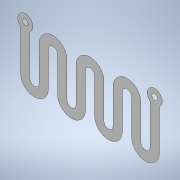
# Autodesk Inventor part: sensor-0002-001
Saved by Autodesk Inventor 2020.1 (Build 241239000, 239)
## iProperties
Created: 2024-03-28
Part Number: sensor-0002-001
Material: Generic
Document SubType Name: Modeling
Designer: MiguelBarbosa
Density: 1 g/cm^3
Appearance: Default
Author: MiguelBarbosa
Autodesk Inventor part; units mm, degrees
ref_plane "YZ Plane" through (0, 0, 0) normal (1, 0, 0) x (0, 1, 0)
ref_plane "XZ Plane" through (0, 0, 0) normal (0, 1, 0) x (-1, 0, 0)
ref_plane "XY Plane" through (0, 0, 0) normal (0, 0, 1) x (1, 0, 0)
sketch "Sketch1" plane through (0, 0, 0) normal (0, 0, 1) x (1, 0, 0)
  circle A0 centre (-2800, 1250) radius 325 construction
  line L0 (-2800, 1250) -> (-2800, -750) construction
  line L1 (-3000, 993.8262) -> (-3000, -750)
  line L2 (-2600, 993.8262) -> (-2600, -750)
  circle A1 centre (-2400, -750) radius 200 construction
  arc A2 (-2600, -750) -> (-2200, -750) centre (-2400, -750) ccw
  circle A3 centre (-2400, -750) radius 600 construction
  arc A4 (-3000, -750) -> (-1800, -750) centre (-2400, -750) ccw
  line L3 (-2200, -750) -> (-2200, 750)
  line L4 (-1800, -750) -> (-1800, 750)
  circle A5 centre (-1600, 750) radius 200 construction
  arc A6 (-1400, 750) -> (-1800, 750) centre (-1600, 750) ccw
  circle A7 centre (-1600, 750) radius 600 construction
  arc A8 (-1000, 750) -> (-2200, 750) centre (-1600, 750) ccw
  line L5 (-1400, 750) -> (-1400, -750)
  line L6 (-1000, 750) -> (-1000, -750)
  circle A9 centre (-800, -750) radius 200 construction
  arc A10 (-1000, -750) -> (-600, -750) centre (-800, -750) ccw
  circle A11 centre (-800, -750) radius 600 construction
  arc A12 (-1400, -750) -> (-200, -750) centre (-800, -750) ccw
  line L7 (-600, -750) -> (-600, 750)
  line L8 (-200, -750) -> (-200, 750)
  arc A13 (600, 750) -> (-600, 750) centre (0, 750) ccw
  arc A14 (200, 750) -> (-200, 750) centre (0, 750) ccw
  line L9 (200, 750) -> (200, -750)
  line L10 (600, 750) -> (600, -750)
  arc A15 (200, -750) -> (1400, -750) centre (800, -750) ccw
  arc A16 (600, -750) -> (1000, -750) centre (800, -750) ccw
  line L11 (1000, -750) -> (1000, 750)
  line L12 (1400, -750) -> (1400, 750)
  arc A17 (2200, 750) -> (1000, 750) centre (1600, 750) ccw
  arc A18 (1800, 750) -> (1400, 750) centre (1600, 750) ccw
  line L13 (1800, 750) -> (1800, -750)
  line L14 (2200, 750) -> (2200, -750)
  arc A19 (1800, -750) -> (3000, -750) centre (2400, -750) ccw
  arc A20 (2200, -750) -> (2600, -750) centre (2400, -750) ccw
  line L15 (2600, -750) -> (2600, 993.8262)
  line L16 (3000, -750) -> (3000, 993.8262)
  circle A21 centre (2800, 1250) radius 325 construction
  arc A22 (-2600, 993.8262) -> (-3000, 993.8262) centre (-2800, 1250) ccw
  arc A23 (3000, 993.8262) -> (2600, 993.8262) centre (2800, 1250) ccw
  circle A24 centre (2800, 1250) radius 125
  circle A25 centre (-2800, 1250) radius 125
  line L17 (-2800, 1250) -> (2800, 1250) construction
  line L18 (-1600, 750) -> (-2400, -750) construction
  point P0 (0, 0)
  point P1 (0, 1250)
  point P2 (-2000, 0)
  dimension "d24" = 400
  dimension "d21" = 200
  dimension "d23" = 2000
  dimension "d25" = 1500
  dimension "d32" = 250
  dimension "d33" = 200
  constraints: 41 horizontal alignment, 38 end point, 36 point on circle, 20 centre point, 18 coincident, 17 vertical, 5 equal radius, 2 midpoint, 2 parallel, 1 vertical alignment, 14 other
  measures "d21" distance between parallel lines of L0 L1
  measures "d23" distance of L0.start L0.end
  measures "d25" distance of L3.start L3.end
  measures "d32" diameter of A25
  measures "d33" radial gap between concentric circles of A25 A0
extrude "Extrusion1" add sketch "Sketch1" along normal mid plane 1
equation "\"d24\" = 2 * d21"
equation "\"d33\" = d21"
body "Solid1"
